Autodesk Fusion 360 part; units mm, degrees
note: some values were not read from the file. Set by a fixed rule: which sketch regions a step uses.
(part 2 of 2)
sketch "Sketch48" plane through (0, 120, 0) normal (0, 1, 0) x (-1, 0, 0)
  line L0 (-219.4869, 85.3819) -> (-209.4869, 95.3819)
  line L1 (-209.4869, 95.3819) -> (-209.4869, 129.2567)
  arc A0 (-209.4869, 129.2567) -> (-209.4869, 41.5071) centre (-199.4869, 85.3819) ccw
  line L2 (-209.4869, 41.5071) -> (-209.4869, 75.3819)
  line L3 (-209.4869, 75.3819) -> (-219.4869, 85.3819)
  circle A1 centre (-199.4869, 85.3819) radius 37.5
  line L4 (-219.4869, 85.3819) -> (-180, 85.3819) construction
  circle A2 centre (-231.9628, 104.1319) radius 5
  line L5 (-199.4869, 85.3819) -> (-231.9628, 104.1319) construction
  circle A3 centre (-231.9628, 66.6319) radius 5
  line L6 (-199.4869, 91.1986) -> (-199.4869, 78) construction
  circle A4 centre (-167.0109, 66.6319) radius 5
  circle A5 centre (-167.0109, 104.1319) radius 5
  dimension "d248" = 75
  dimension "d249" = 10
  dimension "d250" = 30
  constraint concentric A0 A1
  constraint coincident L0.start L3.end
  constraint horizontal L4
  constraint coincident A1 A2.centre
  constraint coincident A0.centre A1.centre
  constraint coincident A2.centre L5.end
  constraint symmetric L4 A2 A3
  constraint perpendicular L4 L6
  constraint symmetric A2 L6 A5
  constraint symmetric A3 L6 A4
  measures "d248" diameter of A1
  measures "d249" diameter of A2
  measures "d250" angle of L4 L5
extrude "Extrude23" cut sketch "Sketch48" against normal up to surface (20 mm away) contours A1 A5 | A1 A5 | A1 A2 | A1 A2 | A1 A3 | A1 A3 | A1 A4 | A1 A4 bodies 14
ref_plane "WorkPlane23" through (0, 0, 0) normal (1, 0, 0) x (0, 1, 0)
copy_body "Body->Comp13" bodies 14 removing the originals makes body 15 in component "Component''''''"
copy_body "Body->Comp14" bodies 1 removing the originals makes body 16 in component "Component'''''''"
copy_body "Body->Comp15" bodies 2 removing the originals makes body 17 in component "Component''''''''"
sketch "Sketch49" plane through (0, 0, 0) normal (1, 0, 0) x (0, 1, 0)
  circle A0 centre (27.6357, 43.8274) radius 10.0037
extrude "Extrude24" add sketch "Sketch49" along normal blind 5 separate body makes body 18
copy_body "Body->Comp16" bodies 18 removing the originals makes body 19 in component "Component'''''''''"
component "Component" placed x (1, 0, 0) y (0, -1, 0) z (0, 0, -1) at (-602.1328, 69.7422, -136.7995)
component "Component'" placed x (1, 0, 0) y (0, 1, 0) z (0, 0, 1) at (-330.0331, 64.7422, 70.7277)
component "Component''" placed x (0.998835, 0, -0.048259) y (0, 1, 0) z (0.048259, 0, 0.998835) at (-264.2285, 69.7422, 69.2707)
component "Component'''" placed x (0.991267, 0, 0.131872) y (0, 1, 0) z (-0.131872, 0, 0.991267) at (-393.1031, 74.7422, 62.5028)
component "Component''''" placed x (1, 0, 0) y (0, 1, 0) z (0, 0, 1) at (-211.5706, -17.7857, -19.8153)
component "Component''''''" placed x (0.984808, 0.173648, 0) y (0, 0, 1) z (0.173648, -0.984808, 0) at (-462.0955, 703.271, -44.2723)
component "Component'''''''" placed x (1, 0, 0) y (0, 0, 1) z (0, -1, 0) at (-300.8451, 592.0784, -49.2723)
component "Component''''''''" placed x (1, 0, 0) y (0, 0, -1) z (0, 1, 0) at (-11.9683, -120.3002, -49.2723)
component "Component'''''''''" placed x (0, 0, -1) y (0, -1, 0) z (-1, 0, 0) at (-215.097, 269.8779, -44.2723)
component "Component'''''" placed x (1, 0, 0) y (0, 1, 0) z (0, 0, 1) at (-194.1192, 87.5279, 67.2097) in component "Component''''"
